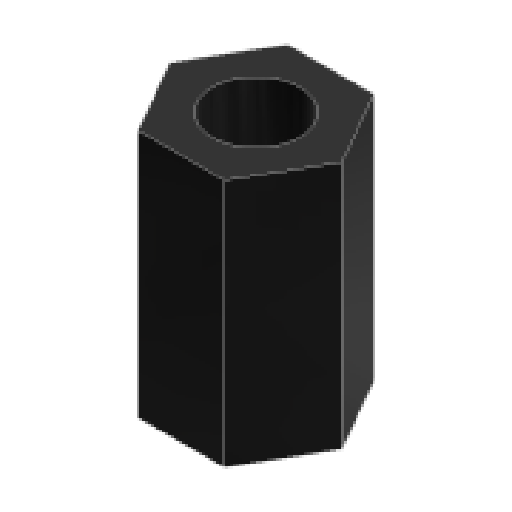
# Autodesk Inventor part: Heated Bed Spacer
Saved by Autodesk Inventor 2023.2 (Build 272271000, 271)
## iProperties
Created: 2023-02-02
Part Number: Heated Bed Spacer
Material: ABS Plastic
Document SubType Name: Modeling
Designer: remop
Density: 1.06 g/cm^3
Appearance: Smooth - Black
Author: remop
Autodesk Inventor part; units mm, degrees
ref_plane "YZ Plane" through (0, 0, 0) normal (1, 0, 0) x (0, 1, 0)
ref_plane "XZ Plane" through (0, 0, 0) normal (0, 1, 0) x (-1, 0, 0)
ref_plane "XY Plane" through (0, 0, 0) normal (0, 0, 1) x (1, 0, 0)
sketch "Sketch1" plane through (0, 0, 0) normal (0, 1, 0) x (-1, 0, 0)
  circle A0 centre (0, 0) radius 1.75
  line L0 (3.4641, 0) -> (1.7321, -3)
  line L1 (1.7321, -3) -> (-1.7321, -3)
  line L2 (-1.7321, -3) -> (-3.4641, 0)
  line L3 (-3.4641, 0) -> (-1.7321, 3)
  line L4 (-1.7321, 3) -> (1.7321, 3)
  line L5 (1.7321, 3) -> (3.4641, 0)
  point P0 (0, -3)
  point P1 (0, 3)
  dimension "d0" = 3.5
  dimension "d1" = 6
  constraints: 12 end point, 2 coincident, 2 midpoint, 1 centre point, 1 horizontal alignment, 13 other
  measures "d0" diameter of A0
  measures "d1" distance from line of L1 point (0, 3)
extrude "Extrusion1" add sketch "Sketch1" along normal blind 10
body "Solid1"
